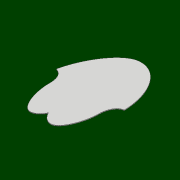
# Autodesk Inventor part: Part2
Saved by Autodesk Inventor 2018 (Build 220112000, 112)
## iProperties
Created: 2021-12-12
Part Number: Part2
Material: 一般
Document SubType Name: Modeling
Designer: gisen
Density: 1 g/cm^3
Appearance: 既定
Author: gisen
Autodesk Inventor part; units mm, degrees
ref_plane "YZ Plane" through (0, 0, 0) normal (1, 0, 0) x (0, 1, 0)
ref_plane "XZ Plane" through (0, 0, 0) normal (0, 1, 0) x (-1, 0, 0)
ref_plane "XY Plane" through (0, 0, 0) normal (0, 0, 1) x (1, 0, 0)
sketch "スケッチ1" plane through (0, 0, 0) normal (0, 0, 1) x (1, 0, 0)
  line L0 (90.7634, 155.7099) -> (92.0352, 158.7983)
  line L1 (92.0352, 158.7983) -> (93.1924, 161.9957)
  line L2 (93.1924, 161.9957) -> (94.231, 165.2798)
  line L3 (94.231, 165.2798) -> (95.1469, 168.6284)
  line L4 (95.1469, 168.6284) -> (95.9357, 172.0191)
  line L5 (95.9357, 172.0191) -> (96.5926, 175.4298)
  line L6 (96.5926, 175.4298) -> (97.1128, 178.8382)
  line L7 (97.1128, 178.8382) -> (97.4912, 182.2221)
  line L8 (97.4912, 182.2221) -> (97.7225, 185.5598)
  line L9 (97.7225, 185.5598) -> (97.7993, 188.7607)
  line L10 (97.7993, 188.7607) -> (97.9539, 192.3082)
  line L11 (97.9539, 192.3082) -> (98.3949, 195.6443)
  line L12 (98.3949, 195.6443) -> (99.1036, 198.7948)
  line L13 (99.1036, 198.7948) -> (100.0567, 201.7172)
  line L14 (100.0567, 201.7172) -> (101.2288, 204.3688)
  line L15 (101.2288, 204.3688) -> (102.5913, 206.7078)
  line L16 (102.5913, 206.7078) -> (104.1122, 208.6948)
  line L17 (104.1122, 208.6948) -> (105.7559, 210.296)
  line L18 (105.7559, 210.296) -> (107.4873, 211.4883)
  line L19 (107.4873, 211.4883) -> (109.3848, 212.3071)
  line L20 (109.3848, 212.3071) -> (112.2448, 213.1939)
  line L21 (112.2448, 213.1939) -> (112.0599, 216.9583)
  line L22 (112.0599, 216.9583) -> (111.5403, 222.8048)
  line L23 (111.5403, 222.8048) -> (110.7528, 228.5509)
  line L24 (110.7528, 228.5509) -> (109.704, 234.1698)
  line L25 (109.704, 234.1698) -> (108.4, 239.6423)
  line L26 (108.4, 239.6423) -> (106.8465, 244.9494)
  line L27 (106.8465, 244.9494) -> (105.0492, 250.0718)
  line L28 (105.0492, 250.0718) -> (103.0134, 254.9902)
  line L29 (103.0134, 254.9902) -> (100.7444, 259.6854)
  line L30 (100.7444, 259.6854) -> (98.2473, 264.1378)
  line L31 (98.2473, 264.1378) -> (95.526, 268.3291)
  line L32 (95.526, 268.3291) -> (92.5539, 272.2662)
  line L33 (92.5539, 272.2662) -> (89.4149, 275.8109)
  line L34 (89.4149, 275.8109) -> (86.1212, 278.952)
  line L35 (86.1212, 278.952) -> (82.6841, 281.679)
  line L36 (82.6841, 281.679) -> (79.1157, 283.9801)
  line L37 (79.1157, 283.9801) -> (75.429, 285.8431)
  line L38 (75.429, 285.8431) -> (71.6392, 287.2546)
  line L39 (71.6392, 287.2546) -> (67.7633, 288.2017)
  line L40 (67.7633, 288.2017) -> (63.8209, 288.6725)
  line L41 (63.8209, 288.6725) -> (59.8891, 288.6571)
  line L42 (59.8891, 288.6571) -> (59.6008, 288.6369)
  line L43 (59.6008, 288.6369) -> (59.3633, 288.6171)
  line L44 (59.3633, 288.6171) -> (59.1237, 288.5943)
  line L45 (59.1237, 288.5943) -> (58.8819, 288.5683)
  line L46 (58.8819, 288.5683) -> (58.6381, 288.5393)
  line L47 (58.6381, 288.5393) -> (58.3925, 288.5071)
  line L48 (58.3925, 288.5071) -> (58.1453, 288.4721)
  line L49 (58.1453, 288.4721) -> (57.8962, 288.434)
  line L50 (57.8962, 288.434) -> (57.6455, 288.393)
  line L51 (57.6455, 288.393) -> (57.3329, 288.3386)
  line L52 (57.3329, 288.3386) -> (54.4137, 287.6123)
  line L53 (54.4137, 287.6123) -> (51.4191, 286.4721)
  line L54 (51.4191, 286.4721) -> (48.4196, 284.9516)
  line L55 (48.4196, 284.9516) -> (45.4214, 283.0662)
  line L56 (45.4214, 283.0662) -> (42.4306, 280.8286)
  line L57 (42.4306, 280.8286) -> (39.4535, 278.2495)
  line L58 (39.4535, 278.2495) -> (36.4974, 275.3388)
  line L59 (36.4974, 275.3388) -> (33.5703, 272.1057)
  line L60 (33.5703, 272.1057) -> (30.6807, 268.5589)
  line L61 (30.6807, 268.5589) -> (27.8382, 264.7077)
  line L62 (27.8382, 264.7077) -> (25.1407, 260.6983)
  line L63 (25.1407, 260.6983) -> (22.5648, 256.513)
  line L64 (22.5648, 256.513) -> (20.1171, 252.1684)
  line L65 (20.1171, 252.1684) -> (17.8051, 247.6819)
  line L66 (17.8051, 247.6819) -> (15.6362, 243.0707)
  line L67 (15.6362, 243.0707) -> (13.6181, 238.3523)
  line L68 (13.6181, 238.3523) -> (11.7584, 233.5439)
  line L69 (11.7584, 233.5439) -> (10.0649, 228.6627)
  line L70 (10.0649, 228.6627) -> (8.5454, 223.7261)
  line L71 (8.5454, 223.7261) -> (7.2127, 218.7693)
  line L72 (7.2127, 218.7693) -> (6.3994, 215.5088)
  line L73 (6.3994, 215.5088) -> (9.3953, 214.1599)
  line L74 (9.3953, 214.1599) -> (10.867, 213.3951)
  line L75 (10.867, 213.3951) -> (12.3084, 212.415)
  line L76 (12.3084, 212.415) -> (13.7316, 211.1582)
  line L77 (13.7316, 211.1582) -> (15.1036, 209.5823)
  line L78 (15.1036, 209.5823) -> (16.3891, 207.6402)
  line L79 (16.3891, 207.6402) -> (17.548, 205.2826)
  line L80 (17.548, 205.2826) -> (18.5357, 202.461)
  line L81 (18.5357, 202.461) -> (19.3035, 199.1294)
  line L82 (19.3035, 199.1294) -> (19.8012, 195.2456)
  line L83 (19.8012, 195.2456) -> (19.9807, 190.7099)
  line L84 (19.9807, 190.7099) -> (20.0542, 187.5056)
  line L85 (20.0542, 187.5056) -> (20.2743, 184.1401)
  line L86 (20.2743, 184.1401) -> (20.6331, 180.7044)
  line L87 (20.6331, 180.7044) -> (21.1244, 177.2262)
  line L88 (21.1244, 177.2262) -> (21.7425, 173.7332)
  line L89 (21.7425, 173.7332) -> (22.4817, 170.2535)
  line L90 (22.4817, 170.2535) -> (23.3366, 166.8152)
  line L91 (23.3366, 166.8152) -> (24.302, 163.4464)
  line L92 (24.302, 163.4464) -> (25.3732, 160.175)
  line L93 (25.3732, 160.175) -> (26.5458, 157.0282)
  line L94 (26.5458, 157.0282) -> (27.8457, 153.9703)
  line L95 (27.8457, 153.9703) -> (29.2115, 151.1647)
  line L96 (29.2115, 151.1647) -> (30.6365, 148.622)
  line L97 (30.6365, 148.622) -> (32.1158, 146.3515)
  line L98 (32.1158, 146.3515) -> (33.6478, 144.3624)
  line L99 (33.6478, 144.3624) -> (35.235, 142.6647)
  line L100 (35.235, 142.6647) -> (36.8865, 141.272)
  line L101 (36.8865, 141.272) -> (38.6171, 140.2083)
  line L102 (38.6171, 140.2083) -> (40.4392, 139.518)
  line L103 (40.4392, 139.518) -> (42.2741, 139.2786)
  line L104 (42.2741, 139.2786) -> (44.1468, 139.416)
  line L105 (44.1468, 139.416) -> (45.9289, 139.81)
  line L106 (45.9289, 139.81) -> (47.6605, 140.4527)
  line L107 (47.6605, 140.4527) -> (49.3299, 141.3299)
  line L108 (49.3299, 141.3299) -> (50.9307, 142.4279)
  line L109 (50.9307, 142.4279) -> (52.4595, 143.735)
  line L110 (52.4595, 143.735) -> (53.9147, 145.2417)
  line L111 (53.9147, 145.2417) -> (55.2951, 146.9407)
  line L112 (55.2951, 146.9407) -> (56.5994, 148.8263)
  line L113 (56.5994, 148.8263) -> (57.8204, 150.8848)
  line L114 (57.8204, 150.8848) -> (57.8769, 150.9927)
  line L115 (57.8769, 150.9927) -> (57.9678, 151.1663)
  line L116 (57.9678, 151.1663) -> (58.1108, 151.4397)
  line L117 (58.1108, 151.4397) -> (58.1996, 151.6095)
  line L118 (58.1996, 151.6095) -> (59.0927, 149.9239)
  line L119 (59.0927, 149.9239) -> (60.4517, 147.7502)
  line L120 (60.4517, 147.7502) -> (61.9067, 145.7852)
  line L121 (61.9067, 145.7852) -> (63.4537, 144.0368)
  line L122 (63.4537, 144.0368) -> (65.0897, 142.5148)
  line L123 (65.0897, 142.5148) -> (66.8115, 141.2308)
  line L124 (66.8115, 141.2308) -> (68.615, 140.1997)
  line L125 (68.615, 140.1997) -> (70.493, 139.4395)
  line L126 (70.493, 139.4395) -> (72.4323, 138.9701)
  line L127 (72.4323, 138.9701) -> (74.4469, 138.8075)
  line L128 (74.4469, 138.8075) -> (76.3205, 139.0249)
  line L129 (76.3205, 139.0249) -> (78.1776, 139.6559)
  line L130 (78.1776, 139.6559) -> (79.9589, 140.6449)
  line L131 (79.9589, 140.6449) -> (81.6683, 141.9544)
  line L132 (81.6683, 141.9544) -> (83.3156, 143.5616)
  line L133 (83.3156, 143.5616) -> (84.9087, 145.4536)
  line L134 (84.9087, 145.4536) -> (86.4511, 147.6213)
  line L135 (86.4511, 147.6213) -> (87.943, 150.0579)
  line L136 (87.943, 150.0579) -> (89.3819, 152.7563)
  line L137 (89.3819, 152.7563) -> (90.7634, 155.7099)
  point P0 (0, 0)
  constraints: 276 end point
extrude "押し出し1" add sketch "スケッチ1" along normal blind 1
